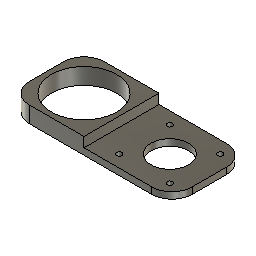
motor mount screw v2 (Autodesk Fusion 360 design; units mm, degrees)
Autodesk Fusion 360 part; units mm, degrees
sketch "Skizze1" plane through (0, 0, 0) normal (0, 0, 1) x (1, 0, 0)
  circle A0 centre (0, 0) radius 20
  line L0 (85, 23) -> (-23, 23)
  line L1 (-23, -23) -> (85, -23)
  line L2 (85, -23) -> (85, 23)
  line L3 (85, 23) -> (-23, -6.2235) construction
  line L4 (-23, 6.2235) -> (85, -23) construction
  line L5 (-23, -23) -> (-23, 23)
  line L6 (37.1516, -15.5) -> (68.1516, 15.5) construction
  line L7 (68.1516, -15.5) -> (37.1516, 15.5) construction
  circle A1 centre (37.1516, 15.5) radius 1.65
  circle A2 centre (37.1516, -15.5) radius 1.65
  circle A3 centre (68.1516, -15.5) radius 1.65
  circle A4 centre (68.1516, 15.5) radius 1.65
  circle A5 centre (52.6516, 0) radius 11.5
  line L8 (68.1516, 15.5) -> (66.5016, 15.5)
  line L9 (38.8016, 15.5) -> (37.1516, 15.5)
  line L10 (68.1516, -15.5) -> (68.1516, -13.85)
  line L11 (68.1516, 13.85) -> (68.1516, 15.5)
  line L12 (37.1516, -15.5) -> (38.8016, -15.5)
  line L13 (66.5016, -15.5) -> (68.1516, -15.5)
  line L14 (37.1516, 15.5) -> (37.1516, 13.85)
  line L15 (37.1516, -13.85) -> (37.1516, -15.5)
  line L16 (20, 0) -> (64, 0)
  point P0 (52.6516, 0)
  dimension "d1" = 31
  dimension "d2" = 31
  dimension "d3" = 3.3
  dimension "d4" = 3.3
  dimension "d5" = 3.3
  dimension "d6" = 3.3
  dimension "d7" = 23
  constraint coincident A0.centre origin
  constraint horizontal L0
  constraint parallel L0 L1
  constraint coincident L3 A0.centre
  constraint coincident L4 A0.centre
  constraint perpendicular L0 L5
  constraint coincident L5 L3.end
  constraint coincident L5 L4.start
  constraint horizontal L12
  constraint perpendicular L10 L12
  constraint parallel L8 L12
  constraint parallel L10 L14
  constraint coincident L6 P0
  constraint coincident L7 P0
  constraint coincident L7.end A1.centre
  constraint coincident L6.start A2.centre
  constraint coincident L7.start A3.centre
  constraint coincident L6.end A4.centre
  constraint coincident P0 A5.centre
  constraint coincident A4 L8.end
  constraint collinear L8 L9
  constraint coincident A1 L9.start
  constraint coincident A3 L10.end
  constraint coincident A4 L11.start
  constraint collinear L10 L11
  constraint coincident A3 L13.start
  constraint collinear L12 L13
  constraint coincident A2 L12.end
  constraint collinear L14 L15
  constraint coincident A2 L15.start
  constraint coincident A1 L14.end
  constraint coincident A0 L16.start
  constraint horizontal L16
  measures "d1" distance of L6.end L7.end
  measures "d2" distance of L7.start L6.end
  measures "d3" diameter of A1
  measures "d4" diameter of A2
  measures "d5" diameter of A3
  measures "d6" diameter of A4
  measures "d7" diameter of A5
extrude "Extrusion1" add sketch "Skizze1" along normal blind 4
sketch "Skizze2" plane through (0, 0, 4) normal (0, 0, 1) x (-1, 0, 0)
  circle A0 centre (-37.1516, 15.5) radius 1.65
  circle A1 centre (0, 0) radius 20
  circle A2 centre (-68.1516, 15.5) radius 1.65
  circle A3 centre (-37.1516, -15.5) radius 1.65
  circle A4 centre (-68.1516, -15.5) radius 1.65
  circle A5 centre (-52.6516, 0) radius 11.5
  line L0 (-85, 23) -> (-85, -23)
  line L1 (-85, -23) -> (23, -23)
  line L2 (23, -23) -> (23, 23)
  line L3 (23, 23) -> (-85, 23)
  line L4 (23, 23) -> (-23, 23)
  line L5 (-23, 23) -> (-23, -23)
  line L6 (-23, -23) -> (23, -23)
  line L7 (23, -23) -> (23, 23)
  line L8 (23, 23) -> (-23, -23) construction
  line L9 (-23, 23) -> (23, -23) construction
  constraint horizontal L4
  constraint perpendicular L4 L5
  constraint parallel L4 L6
  constraint parallel L5 L7
  constraint coincident L8 A1.centre
  constraint coincident L9 A1.centre
  constraint coincident L2.end L3.start
  constraint coincident A1.centre origin
extrude "Extrusion2" add sketch "Skizze2" along normal blind 6 contours L1 L2 L3 L4 L5 L6 L7
extrude "Extrusion3" cut 1 faces at (85, -7.6667, 1.3333) along direction (-1, 0, 0) blind 8
fillet "Abrundung1" radius 12.5 4 edges at (-23, 23, 5) (-23, -23, 5) (77, 23, 2) (77, -23, 2)
